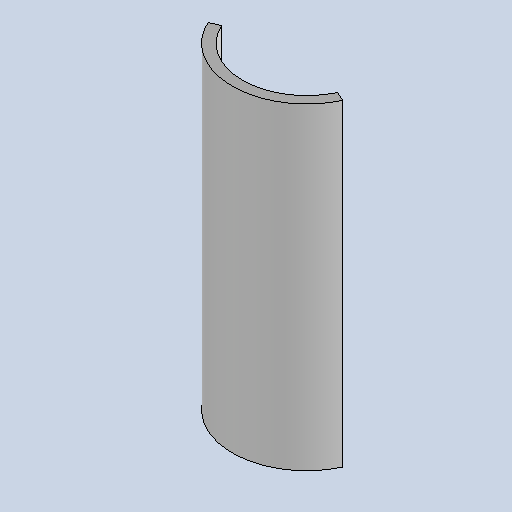
# Autodesk Inventor part: NVPH-303 second tube half
Saved by Autodesk Inventor 2025 (Build 290162010, 162A)
## iProperties
Created: 2024-12-03
Part Number: NVPH-303 second tube half
Material: Generic
Document SubType Name: Modeling
Designer: user
Density: 1 g/cm^3
Appearance: Default
Author: user
Autodesk Inventor part; units mm, degrees
ref_plane "YZ Plane" through (0, 0, 0) normal (1, 0, 0) x (0, 1, 0)
ref_plane "XZ Plane" through (0, 0, 0) normal (0, 1, 0) x (-1, 0, 0)
ref_plane "XY Plane" through (0, 0, 0) normal (0, 0, 1) x (1, 0, 0)
sketch "Sketch1" plane through (0, 0, 0) normal (0, 0, 1) x (1, 0, 0)
  circle A0 centre (0, 0) radius 62.5
  circle A1 centre (0, 0) radius 72.5
  dimension "d1" = 125
  dimension "d6" = 10
  constraints: 2 centre point, 2 coincident
  measures "d1" diameter of A0
  measures "d6" radial gap between concentric circles of A0 A1
extrude "Extrusion1" add sketch "Sketch1" along normal blind 310
sketch "Sketch5" plane through (0, 0, 0) normal (0, 0, 1) x (1, 0, 0)
  circle A0 centre (0, 0) radius 72.5 projected
  circle A1 centre (0, 0) radius 62.5 projected
  line L0 (0, 0) -> (-65.7073, -30.6398)
  line L1 (0, 0) -> (65.7073, -30.6398)
  line L2 (0, 0) -> (0, -72.5) construction
  point P0 (56.6442, -26.4136)
  point P1 (-56.6442, -26.4136)
  dimension "d8" = 130
  constraints: 6 end point, 3 point on circle, 1 vertical, 1 other
  measures "d8" angle of L1 L0
extrude "Extrusion3" cut sketch "Sketch5" along normal through all contours A0 L1 A1 L0 picked at (-11.0811, 68.0627)
body "Solid1"
